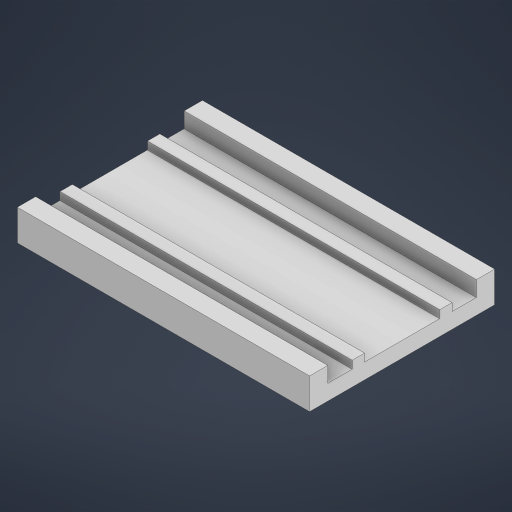
# Autodesk Inventor part: RD53a Gluing Form V1
Saved by Autodesk Inventor 2024 (Build 280153000, 153)
## iProperties
Created: 2023-07-05
Part Number: RD53a Gluing Form V1
Material: Generic
Document SubType Name: Modeling
Designer: Caleb Fangmeier
Density: 1 g/cm^3
Appearance: Default
Author: Caleb Fangmeier
Autodesk Inventor part; units mm, degrees
ref_plane "YZ Plane" through (0, 0, 0) normal (1, 0, 0) x (0, 1, 0)
ref_plane "XZ Plane" through (0, 0, 0) normal (0, 1, 0) x (-1, 0, 0)
ref_plane "XY Plane" through (0, 0, 0) normal (0, 0, 1) x (1, 0, 0)
sketch "Sketch1" plane through (0, 0, 0) normal (0, 1, 0) x (-1, 0, 0)
  line L0 (-30, -19) -> (30, -19)
  line L1 (30, -19) -> (30, 19)
  line L2 (30, 19) -> (-30, 19)
  line L3 (-30, 19) -> (-30, -19)
  line L4 (-30, -19) -> (30, 19) construction
  line L5 (30, -19) -> (-30, 19) construction
  point P0 (0, 0)
  dimension "d0" = 38
  dimension "d1" = 60
  constraints: 12 end point, 2 midpoint, 2 parallel, 1 horizontal, 1 perpendicular
  measures "d0" distance of L0.end L1.end
  measures "d1" distance of L0.start L0.end
extrude "Extrusion1" add sketch "Sketch1" along normal blind 6.35
sketch "Sketch2" plane through (0, 6.35, 0) normal (0, 1, 0) x (1, 0, 0)
  line L0 (-30, 19) -> (-30, -19) projected
  line L1 (30, 15.25) -> (-30, 15.25)
  line L2 (-30, 15.25) -> (-30, -15.25)
  line L3 (-30, -15.25) -> (30, -15.25)
  line L4 (30, -15.25) -> (30, 15.25)
  line L5 (30, 15.25) -> (-30, -15.25) construction
  line L6 (-30, 15.25) -> (30, -15.25) construction
  point P0 (0, 0)
  point P1 (-30, 15.25)
  dimension "d4" = 30.5
  constraints: 12 end point, 2 midpoint, 2 parallel, 1 horizontal, 1 perpendicular, 1 point on line
  measures "d4" distance between parallel lines of L3 L1
extrude "Extrusion2" cut sketch "Sketch2" against normal blind 3.175
sketch "Sketch3" plane through (0, 3.175, 0) normal (0, 1, 0) x (1, 0, 0)
  line L0 (-30, -15.25) -> (-30, 15.25) projected
  line L1 (30, 15.25) -> (30, -15.25) projected
  line L2 (-30, 10.25) -> (30, 10.25)
  line L3 (30, 10.25) -> (30, 7.71)
  line L4 (30, 7.71) -> (-30, 7.71)
  line L5 (-30, 7.71) -> (-30, 10.25)
  line L6 (-30, -7.71) -> (30, -7.71)
  line L7 (30, -7.71) -> (30, -10.25)
  line L8 (30, -10.25) -> (-30, -10.25)
  line L9 (-30, -10.25) -> (-30, -7.71)
  point P0 (0, 0)
  point P1 (30, 10.25)
  point P2 (-30, -10.25)
  point P3 (30, -7.71)
  dimension "d7" = 2.54
  dimension "d8" = 2.54
  dimension "d9" = 20.5
  dimension "d10" = 10.25
  constraints: 16 end point, 4 parallel, 4 point on line, 2 horizontal, 2 perpendicular
  measures "d7" distance between parallel lines of L2 L4
  measures "d8" distance between parallel lines of L6 L8
  measures "d9" distance between parallel lines of L8 L2
  measures "d10" distance from line of L2 point (0, 0)
extrude "Extrusion3" add sketch "Sketch3" along normal blind 1.5875 contours L0 L6 L1 L8 | L0 L2 L1 L4
equation "\"d8\" = d7"
equation "\"d10\" = 0.5 * d9"
body "Solid1"
